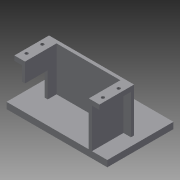
# Autodesk Inventor part: podstawa
Saved by Autodesk Inventor 2013 (Build 170138000, 138)
## iProperties
Created: 2013-03-08
Part Number: podstawa
Material: Generic
Document SubType Name: Modeling
Designer: Masta
Density: 1 g/cm^3
Author: Masta
Autodesk Inventor part; units mm, degrees
ref_plane "YZ Plane" through (0, 0, 0) normal (1, 0, 0) x (0, 1, 0)
ref_plane "XZ Plane" through (0, 0, 0) normal (0, 1, 0) x (-1, 0, 0)
ref_plane "XY Plane" through (0, 0, 0) normal (0, 0, 1) x (1, 0, 0)
sketch "Sketch1" plane through (0, 0, 0) normal (0, 0, 1) x (1, 0, 0)
  line L0 (20.25, 10) -> (-20.25, 10)
  line L1 (-20.25, 10) -> (-20.25, -10)
  line L2 (-20.25, -10) -> (20.25, -10)
  line L3 (20.25, -10) -> (20.25, 10)
  line L4 (20.25, 10) -> (-20.25, -10) construction
  line L5 (-20.25, 10) -> (20.25, -10) construction
  line L6 (-27, 10) -> (-27, 6.25)
  line L7 (27, -10) -> (27, -6.25)
  line L8 (27, 10) -> (-27, -10) construction
  line L9 (-27, 10) -> (27, -10) construction
  line L10 (20.25, -10) -> (27, -10)
  line L11 (20.25, 10) -> (27, 10)
  line L12 (-20.25, 10) -> (-27, 10)
  line L13 (-20.25, -10) -> (-27, -10)
  line L14 (24.25, 5) -> (-24.25, 5) construction
  line L15 (-24.25, 5) -> (-24.25, -5) construction
  line L16 (-24.25, -5) -> (24.25, -5) construction
  line L17 (24.25, -5) -> (24.25, 5) construction
  line L18 (24.25, 5) -> (-24.25, -5) construction
  line L19 (-24.25, 5) -> (24.25, -5) construction
  circle A0 centre (-24.25, 5) radius 1
  line L20 (-20.25, 0) -> (20.25, 0) construction
  line L21 (0, 10) -> (0, -10) construction
  circle A1 centre (-24.25, -5) radius 1
  circle A2 centre (24.25, 5) radius 1
  circle A3 centre (24.25, -5) radius 1
  line L22 (-27, 3.75) -> (-27, -3.75)
  line L23 (-27, 6.25) -> (-27, 3.75)
  line L24 (-27, -6.25) -> (-27, -10)
  line L25 (-27, -3.75) -> (-27, -6.25)
  line L26 (27, -3.75) -> (27, 3.75)
  line L27 (27, -6.25) -> (27, -3.75)
  line L28 (27, 3.75) -> (27, 6.25)
  line L29 (27, 6.25) -> (27, 10)
  line L30 (-22.25, -10) -> (-22.25, 10)
  line L31 (22.25, -10) -> (22.25, 10)
  line L32 (-27, 10) -> (-27, 12)
  line L33 (-27, 12) -> (27, 12)
  line L34 (27, 12) -> (27, 10)
  point P0 (0, 0)
  point P1 (0, 0)
  point P2 (0, 0)
  dimension "d0" = 40.5
  dimension "d1" = 20
  dimension "d2" = 54
  dimension "d3" = 48.5
  dimension "d4" = 10
  dimension "d6" = 2
  dimension "d7" = 2
  dimension "d8" = 2
  dimension "d9" = 2
  constraints: 70 end point, 33 parallel, 11 midpoint, 10 perpendicular, 9 symmetric about line, 4 centre point, 4 point on line, 2 coincident, 2 collinear, 2 horizontal, 3 other
  measures "d0" distance of L3.start L1.end
  measures "d1" distance of L1.end L1.start
  measures "d2" distance of L7.start L8.end
  measures "d3" distance of L17.start L18.end
  measures "d4" distance of L18.end L14.end
  measures "d6" diameter of A0
  measures "d7" distance between parallel lines of L1 L30
  measures "d8" distance between parallel lines of L31 L3
  measures "d9" distance of L6.start L32.end
extrude "Extrusion1" add sketch "Sketch1" along normal blind 3 contours L11 L31 L10 L3 | L0 L12 L32 L33 L34 L11 | L1 L13 L30 L12 | L11 L29 L28 L26 L27 L7 L10 L31 | L30 L13 L24 L25 L22 L23 L6 L12
extrude "Extrusion2" add sketch "Sketch1" against normal blind 9 contours L11 L31 L10 L3 | L0 L12 L32 L33 L34 L11 | L1 L13 L30 L12
extrude "Extrusion3" add sketch "Sketch1" against normal blind 25 contours L11 L31 L10 L3 | L0 L12 L32 L33 L34 L11
sketch "Sketch2" plane through (0, 0, -25) normal (0, 0, -1) x (-1, 0, 0)
  line L0 (27, 10) -> (27, 12) projected
  line L1 (27, 12) -> (-27, 12) projected
  line L2 (-27, 12) -> (-27, 10) projected
  line L3 (-22.25, -10) -> (-20.25, -10) projected
  line L4 (-32, -10) -> (32, -10)
  line L5 (32, -10) -> (32, 32)
  line L6 (32, 32) -> (-32, 32)
  line L7 (-32, 32) -> (-32, -10)
  point P0 (0, 0)
  dimension "d16" = 20
  dimension "d17" = 5
  dimension "d18" = 5
  constraints: 8 end point, 2 parallel, 1 collinear, 1 horizontal, 1 perpendicular
  measures "d16" distance between parallel lines of L6 L1
  measures "d17" distance between parallel lines of L7 L2
  measures "d18" distance between parallel lines of L5 L0
extrude "Extrusion4" add sketch "Sketch2" along normal blind 4
sketch "Sketch3" plane through (0, 0, -9) normal (0, 0, -1) x (-1, 0, 0)
  line L0 (22.25, 10) -> (20.25, 10) projected
  line L1 (20.25, 10) -> (20.25, -10) projected
  line L2 (22.25, -10) -> (22.25, 10) projected
  line L3 (20.25, 4.4217) -> (22.25, 4.4217)
  point P0 (0, 0)
  constraints: 2 end point, 2 point on line, 1 perpendicular
extrude "Extrusion5" add sketch "Sketch3" along normal up to next
body "Solid1"
